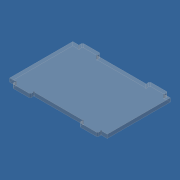
# Autodesk Inventor part: P1704_203
Saved by Autodesk Inventor 2015 (Build 190159000, 159)
## iProperties
Created: 2017-02-08
Part Number: P1704_203
Project: Manette
Material: Plastique PMMA
Description: Paroi latérale- Table
Document SubType Name: Modeling
Designer: Alexandre.PICOTTE
Authority: 80.4x58x3
Density: 1.188 g/cm^3
Appearance: Transparent - Clair
Mass: 15.5108 g
Surface Area: 95.8907 cm^2
Volume: 13.0563 cm^3
Material number: ---
Author: Boris.GAUDARD
Autodesk Inventor part; units mm, degrees
ref_plane "Plan YZ" through (0, 0, 0) normal (1, 0, 0) x (0, 1, 0)
ref_plane "Plan XZ" through (0, 0, 0) normal (0, 1, 0) x (-1, 0, 0)
ref_plane "Plan XY" through (0, 0, 0) normal (0, 0, 1) x (1, 0, 0)
sketch "Esquisse7" plane through (0, 0, 0) normal (0, 0, 1) x (1, 0, 0)
  line L0 (-40.2, -26) -> (-40.2, 26)
  line L1 (-40.2, 26) -> (-35.2, 26)
  line L2 (-35.2, 26) -> (-35.2, 29)
  line L3 (-35.2, 29) -> (-20.2, 29)
  line L4 (-20.2, 29) -> (-20.2, 26)
  line L5 (20.2, 26) -> (20.2, 29)
  line L6 (20.2, 29) -> (35.2, 29)
  line L7 (35.2, 29) -> (35.2, 26)
  line L8 (35.2, 26) -> (40.2, 26)
  line L9 (40.2, 26) -> (40.2, -26)
  line L10 (40.2, -26) -> (35.2, -26)
  line L11 (35.2, -26) -> (35.2, -29)
  line L12 (35.2, -29) -> (20.2, -29)
  line L13 (20.2, -29) -> (20.2, -26)
  line L14 (-20.2, -26) -> (-20.2, -29)
  line L15 (-35.2, -29) -> (-35.2, -26)
  line L16 (-40.2, -26) -> (-35.2, -26)
  line L17 (-35.2, -29) -> (-20.2, -29)
  line L18 (0, -40.6) -> (0, 40.6) construction
  line L19 (-56.28, 0) -> (56.28, 0) construction
  line L20 (-20.2, -26) -> (-7.5, -26)
  line L21 (7.5, -26) -> (20.2, -26)
  line L22 (-20.2, 26) -> (-7.5, 26)
  line L23 (7.5, 26) -> (20.2, 26)
  line L24 (-7.5, -26) -> (7.5, -26)
  line L25 (-7.5, 26) -> (7.5, 26)
  point P0 (0, 0)
  dimension "d33" = 52
  dimension "d34" = 5
  dimension "d35" = 3
  dimension "d36" = 15
  dimension "d51" = 80.4
  constraints: 48 end point, 17 point on line, 10 perpendicular, 6 collinear, 3 parallel, 1 horizontal, 1 vertical, 2 other
  measures "d33" distance of L0.start L0.end
  measures "d34" distance of L0.end L1.end
  measures "d35" distance of L1.end L2.end
  measures "d36" distance of L2.end L3.end
  measures "d51" distance between parallel lines of L9 L0
extrude "Extrusion3" add sketch "Esquisse7" along normal blind 3
chamfer "Chanfrein5" distance 1 angle 45 8 edges at (-20.2, 29, 1.5) (-35.2, 29, 1.5) (20.2, 29, 1.5) (35.2, 29, 1.5) (35.2, -29, 1.5) (20.2, -29, 1.5) (-20.2, -29, 1.5) (-35.2, -29, 1.5)
sketch "Esquisse10" plane through (0, 0, 3) normal (0, 0, 1) x (1, 0, 0)
  line L0 (-34.2, -29) -> (-35.2, -28) construction
  line L1 (-34.2, -29) -> (-21.2, -29) construction
  line L2 (-20.2, -28) -> (-21.2, -29) construction
  line L3 (-20.2, -28) -> (-20.2, -26) construction
  line L4 (-20.2, -26) -> (20.2, -26) construction
  line L5 (20.2, -26) -> (20.2, -28) construction
  line L6 (21.2, -29) -> (20.2, -28) construction
  line L7 (21.2, -29) -> (34.2, -29) construction
  line L8 (35.2, -28) -> (34.2, -29) construction
  line L9 (35.2, -28) -> (35.2, -26) construction
  line L10 (35.2, -26) -> (40.2, -26) construction
  line L11 (40.2, -26) -> (40.2, 26) construction
  line L12 (40.2, 26) -> (35.2, 26) construction
  line L13 (35.2, 26) -> (35.2, 28) construction
  line L14 (34.2, 29) -> (35.2, 28) construction
  line L15 (34.2, 29) -> (21.2, 29) construction
  line L16 (20.2, 28) -> (21.2, 29) construction
  line L17 (20.2, 28) -> (20.2, 26) construction
  line L18 (20.2, 26) -> (-20.2, 26) construction
  line L19 (-20.2, 26) -> (-20.2, 28) construction
  line L20 (-21.2, 29) -> (-20.2, 28) construction
  line L21 (-21.2, 29) -> (-34.2, 29) construction
  line L22 (-35.2, 28) -> (-34.2, 29) construction
  line L23 (-35.2, 28) -> (-35.2, 26) construction
  line L24 (-35.2, 26) -> (-40.2, 26) construction
  line L25 (-40.2, 26) -> (-40.2, -26) construction
  line L26 (-40.2, -26) -> (-35.2, -26) construction
  line L27 (-35.2, -26) -> (-35.2, -28) construction
  point P0 (0, 0)
  constraints: 8 coincident
hole "Perçage4" at (-35.2, 26, 3) at (-20.2, 26, 3) at (20.2, 26, 3) at (35.2, 26, 3) at (-35.2, -26, 3) at (-20.2, -26, 3) at (20.2, -26, 3) at (35.2, -26, 3) direction (0, 0, -1) diameter 1 end through all
